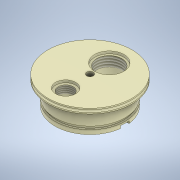
# Autodesk Inventor part: Cuerpo Tapa Sin Paleta
Saved by Autodesk Inventor 2020.3 (Build 243373000, 373)
## iProperties
Created: 2020-06-19
Part Number: Cuerpo Tapa Sin Paleta
Material: Polypropylene
Document SubType Name: Modeling
Designer: Juan
Density: 0.899 g/cm^3
Appearance: Smooth - Ash
Author: Juan
Autodesk Inventor part; units mm, degrees
ref_plane "YZ Plane" through (0, 0, 0) normal (1, 0, 0) x (0, 1, 0)
ref_plane "XZ Plane" through (0, 0, 0) normal (0, 1, 0) x (-1, 0, 0)
ref_plane "XY Plane" through (0, 0, 0) normal (0, 0, 1) x (1, 0, 0)
sketch "Sketch1" plane through (0, 0, 0) normal (0, 0, 1) x (1, 0, 0)
  line L0 (0, 0) -> (0, 33)
  line L1 (0, 33) -> (-50, 33)
  line L2 (0, 0) -> (-41.75, 0)
  line L3 (-41.75, 0) -> (-41.75, 5)
  line L4 (-41.75, 5) -> (-39.5, 5)
  line L5 (-39.5, 5) -> (-39.5, 8.7)
  line L6 (-39.5, 8.7) -> (-41.75, 8.7)
  line L7 (-41.75, 8.7) -> (-26.5, 8.7) construction
  line L8 (-41.75, 8.7) -> (-41.75, 27)
  line L9 (-41.75, 27) -> (-50, 27)
  arc A0 (-50, 28.5) -> (-50, 31.5) centre (-50, 30) ccw
  line L10 (-50, 33) -> (-50, 31.5)
  line L11 (-50, 28.5) -> (-50, 27)
  point P0 (-50, 32.25)
  dimension "d0" = 33
  dimension "d1" = 50
  dimension "d2" = 6
  dimension "d3" = 41.75
  dimension "d4" = 5
  dimension "d5" = 3.7
  dimension "d9" = 39.5
  dimension "d65" = 3
  dimension "d66" = 1.5
  dimension "d67" = 8.25
  constraints: 24 end point, 8 perpendicular, 2 horizontal, 2 point on circle, 2 vertical, 1 centre point, 1 midpoint, 1 point on line, 1 vertical alignment
  measures "d0" distance of L0.start L0.end
  measures "d1" distance of L0.end L1.end
  measures "d2" distance of L1.end L9.end
  measures "d3" distance of L0.start L2.end
  measures "d4" distance of L2.end L3.end
  measures "d5" distance of L4.end L5.end
  measures "d9" distance from line of L0 L4.end
  measures "d65" diameter of A0
  measures "d66" distance of L11.start L9.end
  measures "d67" distance of L8.end L9.end
revolve "Revolution1" add sketch "Sketch1" angle 360 about axis through (0, 0, 0) along (0, 1, 0)
sketch "Sketch3" plane through (0, 33, 0) normal (0, 1, 0) x (1, 0, 0)
  circle A0 centre (0, 0) radius 41
  circle A1 centre (0, 23) radius 16.5 construction
  dimension "d17" = 33
  dimension "d25" = 23
  constraints: 2 centre point, 2 coincident
  measures "d17" diameter of A1
  measures "d25" distance of point (0, 0) A1.centre
hole "Hole1" at (0, 33, -23) direction (0, -1, 0) diameter 30 end through all
sketch "Sketch4" plane through (0, 33, 0) normal (0, 1, 0) x (1, 0, 0)
  circle A0 centre (0, 0) radius 39.5 projected
  point P0 (0, -29)
  dimension "d27" = 29
  constraints: 1 vertical alignment
  measures "d27" distance of point (0, 0) point (0, -29)
hole "Hole2" at (0, 33, 29) direction (0, -1, 0) diameter 18 end through all
sketch "Sketch5" plane through (0, 0, 0) normal (1, 0, 0) x (0, 1, 0)
  line L0 (0, 0) -> (0, 5.05)
  line L1 (0, -41.75) -> (0, 41.75) projected
  line L2 (0, 5.05) -> (3, 5.05)
  line L3 (3, 5.05) -> (3, -5.05)
  line L4 (3, -5.05) -> (0, -5.05)
  line L5 (0, -5.05) -> (0, 0)
  dimension "d35" = 5.05
  dimension "d36" = 3
  dimension "d37" = 10.1
  constraints: 10 end point, 4 perpendicular, 2 point on line
  measures "d35" distance of L0.start L0.end
  measures "d36" distance of L0.end L2.end
  measures "d37" distance of L2.end L3.end
extrude "Extrusion2" cut sketch "Sketch5" against normal through all both and the other way through all
sketch "Sketch6" plane through (0, 33, 0) normal (0, 1, 0) x (1, 0, 0)
  circle A0 centre (0, 23) radius 15 projected
  point P0 (0, 0)
  point P1 (0, 0)
  constraints: 1 coincident
hole "Hole3" at (0, 33, 0) direction (0, -1, 0) diameter 5 end through all
hole "Hole4" at (0, 33, 0) direction (0, -1, 0) diameter 8 depth 20 tip angle 118
sketch "Sketch7" plane through (0, 33, 0) normal (0, 1, 0) x (1, 0, 0)
  circle A0 centre (0, -29) radius 9 projected
  circle A1 centre (0, -29) radius 12
  circle A2 centre (0, 23) radius 15 projected
  circle A3 centre (0, 23) radius 17.5
  point P0 (0, 0)
  dimension "d57" = 24
  dimension "d58" = 35
  constraints: 2 centre point, 2 coincident
  measures "d57" diameter of A1
  measures "d58" diameter of A3
extrude "Extrusion3" cut sketch "Sketch7" against normal blind 3 contours A0 | A1 | A2 | A3
thread "Thread1" size "M20x2" class "6H" standard "ANSI Metric M Profile" length 9
thread "Thread2" size "M33x3" class "6H" standard "ANSI Metric M Profile" length 12
body "Solid1"
